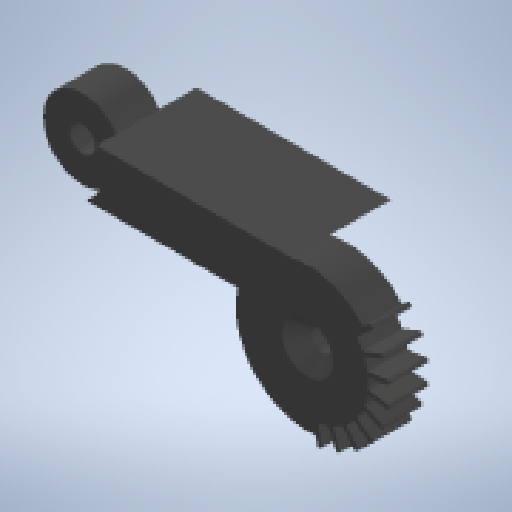
# Autodesk Inventor part: Engrenagem1_0001_001
Saved by Autodesk Inventor 2025.2 (Build 292293000, 293)
## iProperties
Created: 2025-05-31
Part Number: Engrenagem1_0001_001
Material: Borracha
Document SubType Name: Modeling
Designer: Gustavo Sousa
Density: 0.93 g/cm^3
Appearance: Borracha - Preta
Author: Gustavo Sousa
Autodesk Inventor part; units mm, degrees
ref_plane "YZ Plane" through (0, 0, 0) normal (1, 0, 0) x (0, 1, 0)
ref_plane "XZ Plane" through (0, 0, 0) normal (0, 1, 0) x (-1, 0, 0)
ref_plane "XY Plane" through (0, 0, 0) normal (0, 0, 1) x (1, 0, 0)
sketch "Esboço1" plane through (0, 0, 0) normal (0, 0, 1) x (1, 0, 0)
  circle A0 centre (0, 0) radius 5.5
  circle A1 centre (34, -6.8) radius 10 construction
  line L0 (0, 0) -> (0, 5.5) construction
  line L1 (34, -6.8) -> (34, 3.2) construction
  line L2 (4.6595, 2.9222) -> (31.6595, 2.9222)
  line L3 (3.2905, -4.4071) -> (24.2905, -4.4071)
  arc A2 (41.6604, -0.3721) -> (31.6595, 2.9222) centre (34, -6.8) ccw
  circle A3 centre (34, -6.8) radius 8.4
  line L4 (34, -6.8) -> (41.6604, -0.3721) construction
  line L5 (41.6604, -0.3721) -> (42.6563, 0.4635)
  line L6 (42.6563, 0.4635) -> (43.0741, -0.0344)
  line L7 (43.0741, -0.0344) -> (40.8333, -1.9147)
  arc A4 (41.6558, -3.3433) -> (40.8333, -1.9147) centre (34, -6.8) ccw
  arc A5 (43.9789, -6.1508) -> (24.3045, -4.351) centre (34, -6.8) ccw construction
  line L8 (34, -6.8) -> (34, -15.2)
  line L9 (41.6558, -3.3433) -> (34, -6.8) construction
  line L10 (41.6558, -3.3433) -> (44.3664, -2.2436)
  line L11 (44.3664, -2.2436) -> (44.6108, -2.8459)
  line L12 (44.6108, -2.8459) -> (41.9002, -3.9456)
  line L13 (42.2896, -5.4425) -> (45.1925, -5.0818)
  line L14 (45.1925, -5.0818) -> (45.2726, -5.7269)
  line L15 (45.2726, -5.7269) -> (42.3697, -6.0876)
  line L16 (42.3585, -7.6343) -> (45.2558, -8.0372)
  line L17 (45.2558, -8.0372) -> (45.1662, -8.681)
  line L18 (45.1662, -8.681) -> (42.2689, -8.2781)
  line L19 (41.8577, -9.7692) -> (44.552, -10.9083)
  line L20 (44.552, -10.9083) -> (44.2989, -11.507)
  line L21 (44.2989, -11.507) -> (41.6046, -10.3679)
  line L22 (40.8215, -11.7017) -> (43.1292, -13.4993)
  line L23 (43.1292, -13.4993) -> (42.7297, -14.0121)
  line L24 (42.7297, -14.0121) -> (40.4221, -12.2145)
  line L25 (39.3204, -13.3003) -> (41.0842, -15.6339)
  line L26 (41.0842, -15.6339) -> (40.5656, -16.0258)
  line L27 (40.5656, -16.0258) -> (38.8019, -13.6922)
  line L28 (37.4567, -14.4558) -> (38.5564, -17.1664)
  line L29 (38.5564, -17.1664) -> (37.9541, -17.4108)
  line L30 (37.9541, -17.4108) -> (36.8544, -14.7002)
  arc A6 (42.2896, -5.4425) -> (41.9002, -3.9456) centre (34, -6.8) ccw
  line L31 (35.7365, -16.6481) -> (35.9622, -17.9283)
  line L32 (35.9622, -17.9283) -> (35.3221, -18.0412)
  arc A7 (42.3585, -7.6343) -> (42.3697, -6.0876) centre (34, -6.8) ccw
  arc A8 (41.8577, -9.7692) -> (42.2689, -8.2781) centre (34, -6.8) ccw
  arc A9 (40.8215, -11.7017) -> (41.6046, -10.3679) centre (34, -6.8) ccw
  arc A10 (39.3204, -13.3003) -> (40.4221, -12.2145) centre (34, -6.8) ccw
  arc A11 (37.4567, -14.4558) -> (38.8019, -13.6922) centre (34, -6.8) ccw
  line L33 (35.7365, -16.6481) -> (35.4586, -15.0724)
  arc A12 (35.4586, -15.0724) -> (36.8544, -14.7002) centre (34, -6.8) ccw
  line L34 (35.3221, -18.0412) -> (35.0927, -16.7401)
  arc A13 (24.3045, -4.351) -> (35.0927, -16.7401) centre (34, -6.8) ccw
  arc A14 (31.6595, 2.9222) -> (24.3045, -4.351) centre (34, -6.8) ccw
  point P0 (42.1294, -4.6851)
  point P1 (41.2438, -11.0529)
  point P2 (39.8963, -12.7828)
  point P3 (38.1469, -14.105)
  point P4 (36.1645, -14.9163)
  dimension "d17" = 16.8
  dimension "d0" = 11
  dimension "d1" = 20
  dimension "d2" = 34
  dimension "d3" = 6.8
  dimension "d4" = 27
  dimension "d8" = 21
  dimension "d18" = 50
  dimension "d24" = 1.3
  dimension "d25" = 0.65
  dimension "d26" = 90
  dimension "d29" = 90
  dimension "d35" = 15.7
  dimension "d36" = 90
  dimension "d37" = 90
  dimension "d40" = 90
  dimension "d44" = 120
  dimension "d46" = 90
  dimension "d47" = 180
  constraints: 70 end point, 37 point on circle, 14 centre point, 5 concentric, 3 coincident, 3 equal length, 3 vertical, 2 horizontal, 1 collinear, 64 other
  measures "d0" diameter of A0
  measures "d1" diameter of A1
  measures "d2" horizontal distance of point (0, 0) L1.start
  measures "d3" vertical distance of point (0, 0) L1.start
  measures "d4" distance of L2.start L2.end
  measures "d8" distance of L3.start L3.end
  measures "d18" angle of L1 L4
  measures "d24" distance of L4.end L5.end
  measures "d25" distance of L5.end L6.end
  measures "d26" angle of L6 L5
  measures "d29" angle of L6 L7
  measures "d35" angle of L4 L9
  measures "d36" angle of L12 L11
  measures "d37" angle of L11 L10
  measures "d46" angle of L32 L34
  measures "d47" angle of L31 L33
extrude "Extrusão1" add sketch "Esboço1" along normal mid plane 5.45 contours A0 L2 A14 A13 L3
extrude "Extrusão2" add sketch "Esboço1" against normal blind 6 contours A0
extrude "Extrusão3" add sketch "Esboço1" along normal mid plane 5.45 contours A2 L5 L6 L7 A3 L33 L31 L32 L34 A13 A14 | A3 | L10 L11 L12 A3 | A3 L28 L29 L30 | L13 L14 L15 A3 | A3 L25 L26 L27 | L16 L17 L18 A3 | A3 L22 L23 L24 | L19 L20 L21 A3
sketch "Esboço2" plane through (0, 0, -2.725) normal (0, 0, -1) x (-1, 0, 0)
  line L0 (-4.6595, 2.9222) -> (-31.6595, 2.9222) projected
  line L1 (-24.2905, 2.9222) -> (-4.6595, 2.9222)
  arc A0 (-3.2905, -4.4071) -> (-4.6595, 2.9222) centre (0, 0) ccw projected
  arc A1 (-4.6595, 2.9222) -> (-3.2905, -4.4071) centre (0, 0) ccw
  line L2 (-3.2905, -4.4071) -> (-24.2905, -4.4071)
  line L3 (-4.6595, 2.9222) -> (-31.6595, 2.9222)
  line L4 (-24.2905, -4.4071) -> (-3.2905, -4.4071)
  arc A2 (-31.6595, 2.9222) -> (-41.6604, -0.3721) centre (-34, -6.8) ccw projected
  circle A3 centre (-34, -6.8) radius 10 construction
  arc A4 (-24.2905, -4.4071) -> (-31.6595, 2.9222) centre (-34, -6.8) ccw
  dimension "d55" = 5.5
  dimension "d56" = 20
  constraints: 8 end point, 4 point on circle, 3 centre point, 2 collinear, 1 coincident, 1 concentric, 1 point on line
  measures "d55" radius of A1
  measures "d56" diameter of A3
extrude "Extrusão4" add sketch "Esboço2" along normal blind 8.45 contours A1 L2 A4 L0
sketch "Esboço3" plane through (0, 0, 2.725) normal (0, 0, 1) x (1, 0, 0)
  arc A0 (42.3585, -7.6343) -> (42.3697, -6.0876) centre (34, -6.8) ccw projected
  point P0 (0, 0)
  constraints: 1 coincident
hole "Furo1" at (34, -6.8, 2.725) direction (0, 0, -1) diameter 3 end through all countersink diameter 7 countersink angle 90
sketch "Esboço4" plane through (0, 0, 0) normal (0, 0, 1) x (1, 0, 0)
  arc A0 (4.6595, 2.9222) -> (3.2905, -4.4071) centre (0, 0) ccw projected
  constraints: 1 coincident
hole "Furo2" at (0, 0, 0) direction (0, 0, -1) diameter 3.5 end through all
fillet "Arredondamento1" radius 0.25 1 edges at (42.6563, 0.4635, 0)
fillet "Arredondamento2" radius 0.25 1 edges at (43.0741, -0.0344, 0)
fillet "Arredondamento3" radius 0.25 1 edges at (40.8333, -1.9147, 0)
fillet "Arredondamento4" radius 0.25 32 edges at (41.9002, -3.9456, 0) (42.3697, -6.0876, 0) (42.2689, -8.2781, 0) (41.6558, -3.3433, 0) (42.2896, -5.4425, 0) (42.3585, -7.6343, 0) (41.6046, -10.3679, 0) (41.8577, -9.7692, 0) (40.8215, -11.7017, 0) (37.4567, -14.4558, 0) (39.3204, -13.3003, 0) (40.4221, -12.2145, 0) (38.8019, -13.6922, 0) (36.8544, -14.7002, 0) (35.4586, -15.0724, 0) (35.0927, -16.7401, 0) (35.3221, -18.0412, 0) (35.9622, -17.9283, 0) (37.9541, -17.4108, 0) (38.5564, -17.1664, 0) (40.5656, -16.0258, 0) (41.0842, -15.6339, 0) (43.1292, -13.4993, 0) (42.7297, -14.0121, 0) (44.2989, -11.507, 0) (44.552, -10.9083, 0) (45.1662, -8.681, 0) (45.2558, -8.0372, 0) (45.2726, -5.7269, 0) (45.1925, -5.0818, 0) (44.6108, -2.8459, 0) (44.3664, -2.2436, 0)
sketch "Esboço5" plane through (3.2905, -4.4071, 0) normal (0, -1, 0) x (1, 0, 0)
  line L0 (0, 2.725) -> (21, 2.725) projected
  line L1 (21, -1.575) -> (0, -1.575) construction
  line L2 (0, -6) -> (0, 0) projected
  line L3 (21, -2.725) -> (21, 2.725) projected
  line L4 (3.5, -1.575) -> (3.5, -11.175)
  line L5 (21, -11.175) -> (0, -11.175) projected
  line L6 (0, -6) -> (0, -11.175) projected
  line L7 (3.5, -1.575) -> (21, -1.575)
  line L8 (21, -1.575) -> (21, -11.175)
  line L9 (21, -11.175) -> (3.5, -11.175)
  point P0 (-3.2905, 0)
  point P1 (21, -2.725)
  dimension "d69" = 4.3
  dimension "d70" = 3.5
  constraints: 10 end point, 4 point on line, 2 collinear, 1 horizontal, 1 perpendicular, 1 vertical
  measures "d69" distance between parallel lines of L0 L1
  measures "d70" distance between parallel lines of L6 L4
extrude "Extrusão5" cut sketch "Esboço5" against normal blind 1.3
